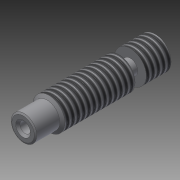
# Autodesk Inventor part: E3D_Heat_Break
Saved by Autodesk Inventor 2014 (Build 180170000, 170)
## iProperties
Created: 2014-09-30
Part Number: E3D_Heat_Break
Material: Generic
Document SubType Name: Modeling
Designer: ThatOtherGuy
Density: 1 g/cm^3
Appearance: Default
Author: ThatOtherGuy
Autodesk Inventor part; units mm, degrees
ref_plane "YZ Plane" through (0, 0, 0) normal (1, 0, 0) x (0, 1, 0)
ref_plane "XZ Plane" through (0, 0, 0) normal (0, 1, 0) x (-1, 0, 0)
ref_plane "XY Plane" through (0, 0, 0) normal (0, 0, 1) x (1, 0, 0)
sketch "Sketch1" plane through (0, 0, 0) normal (0, 0, 1) x (1, 0, 0)
  line L0 (0, 0) -> (0, 10.7581)
  line L1 (1.4, 0) -> (2.1, 0)
  line L2 (2.1, 0) -> (2.4, 0.1732)
  line L3 (2.4, 0.1732) -> (2.4, 4.5)
  line L4 (2.4, 4.5) -> (3, 4.8464)
  line L5 (3, 4.8464) -> (3, 18)
  line L6 (3, 18) -> (1.4, 18)
  line L7 (1.4, 18) -> (1.4, 20.1)
  line L8 (1.4, 20.1) -> (3, 20.1)
  line L9 (3, 20.1) -> (3, 24.7536)
  line L10 (3, 24.7536) -> (2.4, 25.1)
  line L11 (2.4, 25.1) -> (1, 25.1)
  line L12 (1, 25.1) -> (1, 0.4)
  line L13 (1, 0.4) -> (1.4, 0)
  dimension "d0" = 2
  dimension "d1" = 0.4
  dimension "d2" = 0.4
  dimension "d3" = 0.4
  dimension "d4" = 25.1
  dimension "d5" = 20.6
  dimension "d6" = 2.1
  dimension "d7" = 30
  dimension "d8" = 4.2
  dimension "d9" = 4.8
  dimension "d10" = 5
  dimension "d12" = 30
  dimension "d13" = 6
  constraints: 28 end point, 6 parallel, 4 perpendicular, 1 collinear, 1 horizontal alignment, 1 vertical, 1 vertical alignment
  measures "d0" diameter of L12 L0
  measures "d1" distance between parallel lines of L12 L7
  measures "d2" horizontal distance of L1.start L12.end
  measures "d3" horizontal distance of L12.end L1.start
  measures "d4" distance between parallel lines of L11 L1
  measures "d5" distance from line of L11 L3.end
  measures "d6" distance between parallel lines of L8 L6
  measures "d7" angle of L1 L2
  measures "d8" diameter of L1.end L0
  measures "d9" diameter of L3 L0
  measures "d10" distance between parallel lines of L8 L11
  measures "d12" angle of L11 L10
  measures "d13" diameter of L9 L0
revolve "Revolution1" add sketch "Sketch1" angle 360 about axis through (0, 0, 0) along (0, 1, 0)
thread "Thread1" size "M6x1" class "6g" standard "ANSI Metric M Profile" full length
thread "Thread2" size "M6x1" class "6g" standard "ANSI Metric M Profile" full length
equation "\"d3\" = d2"
body "Solid1"
